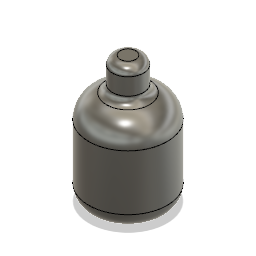
Brenda Bottle (3) (Autodesk Fusion 360 design; units mm, degrees)
Autodesk Fusion 360 part; units mm, degrees
sketch "Sketch1" plane through (0, 0, 0) normal (0, 1, 0) x (1, 0, 0)
  circle A0 centre (0, 0) radius 24.8433
  dimension "d1" = 49.6866
  constraint coincident A0.centre origin
  measures "d1" diameter of A0
extrude "Extrude1" add sketch "Sketch1" along normal blind 60
fillet "Fillet1" radius 10 1 edges at (-23.1621, 0, 8.9837)
fillet "Fillet2" radius 15 1 edges at (-23.1621, 60, 8.9837)
extrude "Extrude2" add 1 faces at (-1.6406, 60, 2.8415) along direction (0, 1, 0) blind 20
fillet "Fillet3" radius 5 1 edges at (-9.1772, 80, 3.5595) 1 faces at (9.8311, 73.3333, 0.4906)
